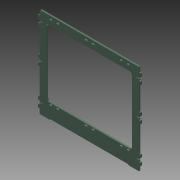
# Autodesk Inventor part: przod_gt2
Saved by Autodesk Inventor 2013 (Build 170138000, 138)
## iProperties
Created: 2014-01-09
Part Number: przod_gt2
Material: Generic
Document SubType Name: Modeling
Designer: dzban
Density: 1 g/cm^3
Author: dzban
Autodesk Inventor part; units mm, degrees
ref_plane "YZ Plane" through (0, 0, 0) normal (1, 0, 0) x (0, 1, 0)
ref_plane "XZ Plane" through (0, 0, 0) normal (0, 1, 0) x (-1, 0, 0)
ref_plane "XY Plane" through (0, 0, 0) normal (0, 0, 1) x (1, 0, 0)
sketch "Sketch1" plane through (0, 0, 0) normal (0, 1, 0) x (-1, 0, 0)
  line L0 (82.0592, -363.263) -> (75.0592, -363.263)
  line L1 (75.0592, -363.263) -> (75.0592, -369.363)
  line L2 (75.0592, -369.363) -> (69.0592, -369.663)
  line L3 (69.0592, -369.663) -> (69.0592, -381.463)
  line L4 (69.0592, -381.463) -> (75.0592, -381.763)
  line L5 (75.0592, -381.763) -> (75.0592, -401.763)
  line L6 (75.0592, -401.763) -> (115.0592, -401.763)
  line L7 (115.0592, -401.763) -> (118.0592, -398.763)
  line L8 (118.0592, -398.763) -> (427.2592, -398.763)
  line L9 (427.2592, -398.763) -> (430.2592, -401.763)
  line L10 (430.2592, -401.763) -> (470.2592, -401.763)
  line L11 (470.2592, -401.763) -> (470.2592, -381.763)
  line L12 (470.2592, -381.763) -> (476.2592, -381.463)
  line L13 (476.2592, -381.463) -> (476.2592, -369.663)
  line L14 (476.2592, -369.663) -> (470.2592, -369.363)
  line L15 (470.2592, -369.363) -> (470.2592, -363.263)
  line L16 (470.2592, -363.263) -> (463.2592, -363.263)
  line L17 (463.2592, -363.263) -> (463.2592, -364.513)
  line L18 (463.2592, -364.513) -> (461.4592, -364.513)
  line L19 (461.4592, -364.513) -> (461.4592, -363.263)
  line L20 (461.4592, -363.263) -> (459.6592, -363.263)
  line L21 (459.6592, -363.263) -> (459.6592, -360.263)
  line L22 (459.6592, -360.263) -> (461.4592, -360.263)
  line L23 (461.4592, -360.263) -> (461.4592, -359.013)
  line L24 (461.4592, -359.013) -> (463.2592, -359.013)
  line L25 (463.2592, -359.013) -> (463.2592, -360.263)
  line L26 (463.2592, -360.263) -> (470.2592, -360.263)
  line L27 (470.2592, -360.263) -> (470.2592, -354.163)
  line L28 (470.2592, -354.163) -> (476.2592, -353.863)
  line L29 (476.2592, -353.863) -> (476.2592, -342.063)
  line L30 (476.2592, -342.063) -> (470.2592, -341.763)
  line L31 (470.2592, -341.763) -> (470.2592, -237.363)
  line L32 (470.2592, -237.363) -> (476.2592, -237.063)
  line L33 (476.2592, -237.063) -> (476.2592, -225.263)
  line L34 (476.2592, -225.263) -> (470.2592, -224.963)
  line L35 (470.2592, -224.963) -> (470.2592, -218.863)
  line L36 (470.2592, -218.863) -> (463.2592, -218.863)
  line L37 (463.2592, -218.863) -> (463.2592, -220.113)
  line L38 (463.2592, -220.113) -> (461.4592, -220.113)
  line L39 (461.4592, -220.113) -> (461.4592, -218.863)
  line L40 (461.4592, -218.863) -> (459.6592, -218.863)
  line L41 (459.6592, -218.863) -> (459.6592, -215.863)
  line L42 (459.6592, -215.863) -> (461.4592, -215.863)
  line L43 (461.4592, -215.863) -> (461.4592, -214.613)
  line L44 (461.4592, -214.613) -> (463.2592, -214.613)
  line L45 (463.2592, -214.613) -> (463.2592, -215.863)
  line L46 (463.2592, -215.863) -> (470.2592, -215.863)
  line L47 (470.2592, -215.863) -> (470.2592, -209.763)
  line L48 (470.2592, -209.763) -> (476.2592, -209.463)
  line L49 (476.2592, -209.463) -> (476.2592, -197.663)
  line L50 (476.2592, -197.663) -> (470.2592, -197.363)
  line L51 (470.2592, -197.363) -> (470.2592, -102.363)
  line L52 (470.2592, -102.363) -> (476.2592, -102.063)
  line L53 (476.2592, -102.063) -> (476.2592, -90.263)
  line L54 (476.2592, -90.263) -> (470.2592, -89.963)
  line L55 (470.2592, -89.963) -> (470.2592, -83.863)
  line L56 (470.2592, -83.863) -> (463.2592, -83.863)
  line L57 (463.2592, -83.863) -> (463.2592, -85.113)
  line L58 (463.2592, -85.113) -> (461.4592, -85.113)
  line L59 (461.4592, -85.113) -> (461.4592, -83.863)
  line L60 (461.4592, -83.863) -> (459.6592, -83.863)
  line L61 (459.6592, -83.863) -> (459.6592, -80.863)
  line L62 (459.6592, -80.863) -> (461.4592, -80.863)
  line L63 (461.4592, -80.863) -> (461.4592, -79.613)
  line L64 (461.4592, -79.613) -> (463.2592, -79.613)
  line L65 (463.2592, -79.613) -> (463.2592, -80.863)
  line L66 (463.2592, -80.863) -> (470.2592, -80.863)
  line L67 (470.2592, -80.863) -> (470.2592, -74.763)
  line L68 (470.2592, -74.763) -> (476.2592, -74.463)
  line L69 (476.2592, -74.463) -> (476.2592, -62.663)
  line L70 (476.2592, -62.663) -> (470.2592, -62.363)
  line L71 (470.2592, -62.363) -> (470.2592, -47.363)
  arc A0 (470.2592, -47.363) -> (465.2592, -42.363) centre (465.2592, -47.363) ccw
  line L72 (465.2592, -42.363) -> (80.0592, -42.363)
  arc A1 (80.0592, -42.363) -> (75.0592, -47.363) centre (80.0592, -47.363) ccw
  line L73 (75.0592, -47.363) -> (75.0592, -62.363)
  line L74 (75.0592, -62.363) -> (69.0592, -62.663)
  line L75 (69.0592, -62.663) -> (69.0592, -74.463)
  line L76 (69.0592, -74.463) -> (75.0592, -74.763)
  line L77 (75.0592, -74.763) -> (75.0592, -80.863)
  line L78 (75.0592, -80.863) -> (82.0592, -80.863)
  line L79 (82.0592, -80.863) -> (82.0592, -79.613)
  line L80 (82.0592, -79.613) -> (83.8592, -79.613)
  line L81 (83.8592, -79.613) -> (83.8592, -80.863)
  line L82 (83.8592, -80.863) -> (85.6592, -80.863)
  line L83 (85.6592, -80.863) -> (85.6592, -83.863)
  line L84 (85.6592, -83.863) -> (83.8592, -83.863)
  line L85 (83.8592, -83.863) -> (83.8592, -85.113)
  line L86 (83.8592, -85.113) -> (82.0592, -85.113)
  line L87 (82.0592, -85.113) -> (82.0592, -83.863)
  line L88 (82.0592, -83.863) -> (75.0592, -83.863)
  line L89 (75.0592, -83.863) -> (75.0592, -89.963)
  line L90 (75.0592, -89.963) -> (69.0592, -90.263)
  line L91 (69.0592, -90.263) -> (69.0592, -102.063)
  line L92 (69.0592, -102.063) -> (75.0592, -102.363)
  line L93 (75.0592, -102.363) -> (75.0592, -197.363)
  line L94 (75.0592, -197.363) -> (69.0592, -197.663)
  line L95 (69.0592, -197.663) -> (69.0592, -209.463)
  line L96 (69.0592, -209.463) -> (75.0592, -209.763)
  line L97 (75.0592, -209.763) -> (75.0592, -215.863)
  line L98 (75.0592, -215.863) -> (82.0592, -215.863)
  line L99 (82.0592, -215.863) -> (82.0592, -214.613)
  line L100 (82.0592, -214.613) -> (83.8592, -214.613)
  line L101 (83.8592, -214.613) -> (83.8592, -215.863)
  line L102 (83.8592, -215.863) -> (85.6592, -215.863)
  line L103 (85.6592, -215.863) -> (85.6592, -218.863)
  line L104 (85.6592, -218.863) -> (83.8592, -218.863)
  line L105 (83.8592, -218.863) -> (83.8592, -220.113)
  line L106 (83.8592, -220.113) -> (82.0592, -220.113)
  line L107 (82.0592, -220.113) -> (82.0592, -218.863)
  line L108 (82.0592, -218.863) -> (75.0592, -218.863)
  line L109 (75.0592, -218.863) -> (75.0592, -224.963)
  line L110 (75.0592, -224.963) -> (69.0592, -225.263)
  line L111 (69.0592, -225.263) -> (69.0592, -237.063)
  line L112 (69.0592, -237.063) -> (75.0592, -237.363)
  line L113 (75.0592, -237.363) -> (75.0592, -341.763)
  line L114 (75.0592, -341.763) -> (69.0592, -342.063)
  line L115 (69.0592, -342.063) -> (69.0592, -353.863)
  line L116 (69.0592, -353.863) -> (75.0592, -354.163)
  line L117 (75.0592, -354.163) -> (75.0592, -360.263)
  line L118 (75.0592, -360.263) -> (82.0592, -360.263)
  line L119 (82.0592, -360.263) -> (82.0592, -359.013)
  line L120 (82.0592, -359.013) -> (83.8592, -359.013)
  line L121 (83.8592, -359.013) -> (83.8592, -360.263)
  line L122 (83.8592, -360.263) -> (85.6592, -360.263)
  line L123 (85.6592, -360.263) -> (85.6592, -363.263)
  line L124 (85.6592, -363.263) -> (83.8592, -363.263)
  line L125 (83.8592, -363.263) -> (83.8592, -364.513)
  line L126 (83.8592, -364.513) -> (82.0592, -364.513)
  line L127 (82.0592, -364.513) -> (82.0592, -363.263)
  line L128 (392.8592, -351.763) -> (392.8592, -345.363)
  line L129 (392.8592, -345.363) -> (404.8592, -345.363)
  line L130 (404.8592, -345.363) -> (404.8592, -351.763)
  line L131 (404.8592, -351.763) -> (392.8592, -351.763)
  line L132 (420.4592, -351.763) -> (420.4592, -345.363)
  line L133 (420.4592, -345.363) -> (432.4592, -345.363)
  line L134 (432.4592, -345.363) -> (432.4592, -351.763)
  line L135 (432.4592, -351.763) -> (420.4592, -351.763)
  line L136 (252.8592, -351.763) -> (252.8592, -345.363)
  line L137 (252.8592, -345.363) -> (264.8592, -345.363)
  line L138 (264.8592, -345.363) -> (264.8592, -351.763)
  line L139 (264.8592, -351.763) -> (252.8592, -351.763)
  line L140 (280.4592, -351.763) -> (280.4592, -345.363)
  line L141 (280.4592, -345.363) -> (292.4592, -345.363)
  line L142 (292.4592, -345.363) -> (292.4592, -351.763)
  line L143 (292.4592, -351.763) -> (280.4592, -351.763)
  line L144 (112.8592, -351.763) -> (112.8592, -345.363)
  line L145 (112.8592, -345.363) -> (124.8592, -345.363)
  line L146 (124.8592, -345.363) -> (124.8592, -351.763)
  line L147 (124.8592, -351.763) -> (112.8592, -351.763)
  line L148 (140.4592, -351.763) -> (140.4592, -345.363)
  line L149 (140.4592, -345.363) -> (152.4592, -345.363)
  line L150 (152.4592, -345.363) -> (152.4592, -351.763)
  line L151 (152.4592, -351.763) -> (140.4592, -351.763)
  line L152 (392.8592, -56.763) -> (392.8592, -50.363)
  line L153 (392.8592, -50.363) -> (404.8592, -50.363)
  line L154 (404.8592, -50.363) -> (404.8592, -56.763)
  line L155 (404.8592, -56.763) -> (392.8592, -56.763)
  line L156 (420.4592, -56.763) -> (420.4592, -50.363)
  line L157 (420.4592, -50.363) -> (432.4592, -50.363)
  line L158 (432.4592, -50.363) -> (432.4592, -56.763)
  line L159 (432.4592, -56.763) -> (420.4592, -56.763)
  line L160 (252.8592, -56.763) -> (252.8592, -50.363)
  line L161 (252.8592, -50.363) -> (264.8592, -50.363)
  line L162 (264.8592, -50.363) -> (264.8592, -56.763)
  line L163 (264.8592, -56.763) -> (252.8592, -56.763)
  line L164 (280.4592, -56.763) -> (280.4592, -50.363)
  line L165 (280.4592, -50.363) -> (292.4592, -50.363)
  line L166 (292.4592, -50.363) -> (292.4592, -56.763)
  line L167 (292.4592, -56.763) -> (280.4592, -56.763)
  line L168 (112.8592, -56.763) -> (112.8592, -50.363)
  line L169 (112.8592, -50.363) -> (124.8592, -50.363)
  line L170 (124.8592, -50.363) -> (124.8592, -56.763)
  line L171 (124.8592, -56.763) -> (112.8592, -56.763)
  line L172 (140.4592, -56.763) -> (140.4592, -50.363)
  line L173 (140.4592, -50.363) -> (152.4592, -50.363)
  line L174 (152.4592, -50.363) -> (152.4592, -56.763)
  line L175 (152.4592, -56.763) -> (140.4592, -56.763)
  arc A2 (442.2592, -85.363) -> (432.2592, -75.363) centre (432.2592, -85.363) ccw
  line L176 (442.2592, -85.363) -> (442.2592, -332.363)
  arc A3 (432.2592, -342.363) -> (442.2592, -332.363) centre (432.2592, -332.363) ccw
  line L177 (432.2592, -342.363) -> (113.0592, -342.363)
  arc A4 (103.0592, -332.363) -> (113.0592, -342.363) centre (113.0592, -332.363) ccw
  line L178 (103.0592, -332.363) -> (103.0592, -85.363)
  arc A5 (113.0592, -75.363) -> (103.0592, -85.363) centre (113.0592, -85.363) ccw
  line L179 (113.0592, -75.363) -> (432.2592, -75.363)
  circle A6 centre (132.6592, -53.563) radius 1.5
  circle A7 centre (272.6592, -53.563) radius 1.5
  circle A8 centre (412.6592, -53.563) radius 1.5
  circle A9 centre (132.6592, -348.563) radius 1.5
  circle A10 centre (272.6592, -348.563) radius 1.5
  circle A11 centre (412.6592, -348.563) radius 1.5
  circle A12 centre (444.1931, -68.563) radius 1.5
  circle A13 centre (84.0592, -100.363) radius 1.5
  circle A14 centre (461.2592, -100.363) radius 1.5
  circle A15 centre (452.2592, -109.363) radius 1.5
  circle A16 centre (93.0592, -109.363) radius 1.5
  circle A17 centre (444.1931, -62.563) radius 1.5
  point P0 (0, 0)
  dimension "d0" = 42.3629
  dimension "d1" = 75.0592
  dimension "d2" = 395.2
  dimension "d3" = 359.4
  dimension "d4" = 3
  dimension "d5" = 40
  dimension "d6" = 135
  dimension "d7" = 40
  dimension "d8" = 5
  dimension "d9" = 33
  dimension "d10" = 28
  dimension "d11" = 56.4
  dimension "d12" = 28
  dimension "d13" = 10
  dimension "d14" = 6.4
  dimension "d15" = 12
  dimension "d16" = 7.8
  dimension "d17" = 7.8
  dimension "d18" = 12
  dimension "d19" = 140
  dimension "d20" = 140
  dimension "d21" = 12
  dimension "d22" = 7.8
  dimension "d23" = 7.8
  dimension "d24" = 12
  dimension "d25" = 12
  dimension "d26" = 7.8
  dimension "d27" = 7.8
  dimension "d28" = 12
  dimension "d29" = 11.2
  dimension "d31" = 3.2
  dimension "d32" = 3
  dimension "d33" = 6.2
  dimension "d34" = 3.2
  dimension "d35" = 6.4
  dimension "d38" = 6
  dimension "d39" = 6
  dimension "d40" = 10.6
  dimension "d41" = 10.6
  dimension "d42" = 197.6
  dimension "d43" = 9
  dimension "d44" = 9
  dimension "d45" = 9
  dimension "d46" = 58
  dimension "d47" = 9
  dimension "d48" = 9
  dimension "d49" = 8.8
  dimension "d50" = 7
  constraints: 360 end point, 150 parallel, 62 collinear, 30 tangent, 25 perpendicular, 18 centre point, 15 equal radius, 12 point on circle, 6 horizontal alignment, 3 vertical alignment, 1 horizontal
  measures "d0" distance from line of point (0, 0) L72
  measures "d1" distance from line of point (0, 0) L73
  measures "d2" distance between parallel lines of L71 L73
  measures "d3" distance between parallel lines of L72 L6
  measures "d4" distance between parallel lines of L8 L6
  measures "d5" distance of L5.end L6.end
  measures "d6" angle of L7 L6
  measures "d7" distance of L9.end L10.end
  measures "d8" radius of A1
  measures "d9" distance between parallel lines of L179 L72
  measures "d10" distance between parallel lines of L178 L93
  measures "d11" distance between parallel lines of L177 L8
  measures "d12" distance between parallel lines of L176 L51
  measures "d13" radius of A2
  measures "d14" distance between parallel lines of L169 L171
  measures "d15" distance between parallel lines of L170 L168
  measures "d16" distance from line of A6.centre L170
  measures "d17" distance from line of L172 A6.centre
  measures "d18" distance between parallel lines of L174 L172
  measures "d19" distance of A7.centre A6.centre
  measures "d20" distance of A8.centre A7.centre
  measures "d21" distance between parallel lines of L162 L160
  measures "d22" distance from line of A7.centre L162
  measures "d23" distance from line of L164 A7.centre
  measures "d24" distance between parallel lines of L166 L164
  measures "d25" distance between parallel lines of L154 L152
  measures "d26" distance from line of A8.centre L154
  measures "d27" distance from line of L156 A8.centre
  measures "d28" distance between parallel lines of L158 L156
  measures "d29" distance from line of L72 A6.centre
  measures "d31" distance from line of L169 A6.centre
  measures "d32" diameter of A6
  measures "d33" distance from line of L177 A9.centre
  measures "d34" distance from line of A9.centre L145
  measures "d35" distance between parallel lines of L145 L147
  measures "d38" distance between parallel lines of L71 L69
  measures "d39" distance between parallel lines of L73 L75
  measures "d40" distance from line of L83.end L89
  measures "d41" distance between parallel lines of L27 L21
  measures "d42" distance from line of A7.centre L73
  measures "d43" horizontal distance of A13.centre A16.centre
  measures "d44" horizontal distance of A13.centre A16.centre
  measures "d45" distance from line of L93 A13.centre
  measures "d46" distance from line of L72 A13.centre
  measures "d47" distance from line of L51 A14.centre
  measures "d48" horizontal distance of A15.centre A14.centre
  measures "d49" distance between parallel lines of L63 L67
  measures "d50" distance between parallel lines of L67 L65
extrude "Extrusion1" add sketch "Sketch1" along normal blind 6
body "Solid1"
